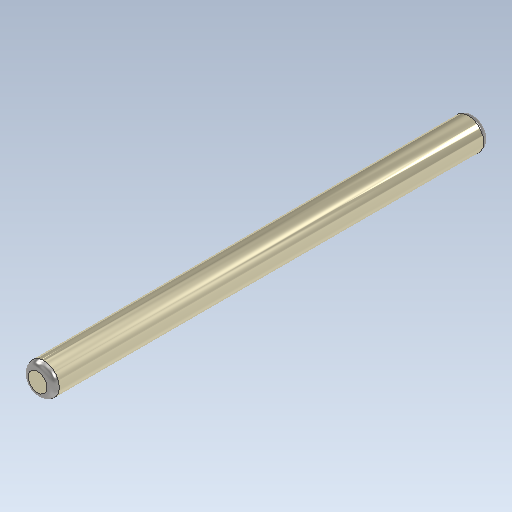
# Autodesk Inventor part: Axle
Saved by Autodesk Inventor 2020 (Build 240168000, 168)
## iProperties
Created: 2019-05-20
Part Number: Axle
Material: Stainless Steel
Document SubType Name: Modeling
Designer: chitl
Density: 8 g/cm^3
Appearance: Semi-Polished
Mass: 22.4225 g
Surface Area: 18.1363 cm^2
Volume: 2.80282 cm^3
Author: chitl
Autodesk Inventor part; units mm, degrees
ref_plane "YZ Plane" through (0, 0, 0) normal (1, 0, 0) x (0, 1, 0)
ref_plane "XZ Plane" through (0, 0, 0) normal (0, 1, 0) x (-1, 0, 0)
ref_plane "XY Plane" through (0, 0, 0) normal (0, 0, 1) x (1, 0, 0)
sketch "Sketch1" plane through (0, 0, 0) normal (0, 0, 1) x (1, 0, 0)
  circle A0 centre (0, 0) radius 3.175
  dimension "d0" = 6.35
  constraints: 1 centre point, 1 coincident
  measures "d0" diameter of A0
extrude "Extrusion1" add sketch "Sketch1" along normal blind 88.9
fillet "Fillet1" radius 1.27 2 edges at (-3.175, 0, 88.9) (-3.175, 0, 0)
body "Solid1"
